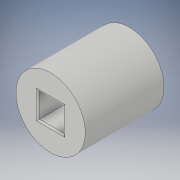
# Autodesk Inventor part: spline coupling
Saved by Autodesk Inventor 2017 (Build 210142000, 142)
## iProperties
Created: 2017-11-16
Part Number: spline coupling
Material: Generic
Document SubType Name: Modeling
Designer: Mitch
Density: 1 g/cm^3
Appearance: Default
Author: Mitch
Autodesk Inventor part; units mm, degrees
ref_plane "YZ Plane" through (0, 0, 0) normal (1, 0, 0) x (0, 1, 0)
ref_plane "XZ Plane" through (0, 0, 0) normal (0, 1, 0) x (-1, 0, 0)
ref_plane "XY Plane" through (0, 0, 0) normal (0, 0, 1) x (1, 0, 0)
sketch "Sketch1" plane through (0, 0, 0) normal (0, 0, 1) x (1, 0, 0)
  circle A0 centre (0, 0) radius 5.588
  dimension "d0" = 11.176
  constraints: 1 centre point, 1 coincident
  measures "d0" diameter of A0
extrude "Extrusion1" add sketch "Sketch1" along normal blind 12.7
sketch "Sketch2" plane through (0, 0, 0) normal (0, 0, -1) x (-1, 0, 0)
  circle A0 centre (0, 0.2754) radius 2.667
  line L0 (0.25, 2.9307) -> (0.0654, 3.4634)
  line L1 (0.0534, 3.4719) -> (-0.0534, 3.4719)
  line L2 (-0.0654, 3.4634) -> (-0.25, 2.9307)
  line L3 (0.25, 2.9307) -> (-0.25, 2.9307)
  line L4 (0, 4.3756) -> (0, 0.2754)
  arc A1 (-0.0534, 3.4719) -> (-0.0654, 3.4634) centre (-0.0534, 3.4592) ccw
  arc A2 (0.0654, 3.4634) -> (0.0534, 3.4719) centre (0.0534, 3.4592) ccw
  point P0 (0, 0)
  point P1 (0.0625, 3.4719)
  point P2 (-0.0625, 3.4719)
  dimension "d3" = 5.334
  dimension "d26" = 0.0625
  dimension "d27" = 0.0625
  dimension "d29" = 0.25
  dimension "d30" = 0.25
  dimension "d31" = 0.5413
  dimension "d32" = 0.0127
  constraints: 10 end point, 4 point on circle, 4 point on line, 4 tangent, 2 centre point, 1 equal radius, 1 horizontal, 1 parallel, 3 other
  measures "d26" distance from line of point (0.062, 3.472) L4
  measures "d27" distance from line of point (-0.062, 3.472) L4
  measures "d29" distance from line of L0.start L4
  measures "d30" distance from line of L2.end L4
  measures "d31" distance between parallel lines of L3 L1
  measures "d32" radius of A1
extrude "Extrusion2" cut sketch "Sketch2" against normal blind 3.81 contours A0 L3 | L3 L4 A0 | A0 L4 L3
sketch "Sketch3" plane through (0, 0, 0) normal (0, 0, -1) x (-1, 0, 0)
  circle A0 centre (0, 0.2754) radius 2.667 projected
  line L0 (0, 0.2754) -> (0, 5.2582)
  line L1 (-0.25, 2.9307) -> (-0.0625, 3.4719)
  line L2 (-0.0625, 3.4719) -> (0.0625, 3.4719)
  line L3 (0.0625, 3.4719) -> (0.25, 2.9307)
  line L4 (-0.25, 2.9307) -> (0.25, 2.9307)
  point P0 (0, 0)
  dimension "d35" = 0.0625
  dimension "d36" = 0.0625
  dimension "d37" = 0.25
  dimension "d38" = 0.5413
  constraints: 10 end point, 2 point on circle, 1 horizontal, 1 parallel, 1 vertical
  measures "d35" distance from line of L2.end L0
  measures "d36" distance from line of L1.end L0
  measures "d37" distance from line of L1.start L0
  measures "d38" distance between parallel lines of L4 L2
extrude "Extrusion3" cut sketch "Sketch3" against normal blind 3.81 contours A0 L0 L2 L3 | L1 L2 L0 A0
pattern_circular "Circular Pattern1" count 23 over 360 about axis through (0, 0.2754, 0) along (0, 0, 1) of "Extrusion3"
fillet "Fillet1" radius 0.254 23 edges at (-1.0625, 2.7216, 0) (-0.3632, 2.9176, 0) (0.3632, 2.9176, 0) (1.0625, 2.7216, 0) (1.6831, 2.3442, 0) (2.1789, 1.8134, 0) (2.513, 1.1685, 0) (2.6608, 0.4574, 0) (2.6112, -0.2672, 0) (2.368, -0.9516, 0) (1.9491, -1.545, 0) (1.3857, -2.0033, 0) (0.7195, -2.2927, 0) (0, -2.3916, 0) (-0.7195, -2.2927, 0) (-1.3857, -2.0033, 0) (-1.9491, -1.545, 0) (-2.368, -0.9516, 0) (-2.6112, -0.2672, 0) (-2.6608, 0.4574, 0) (-2.513, 1.1685, 0) (-2.1789, 1.8134, 0) (-1.6831, 2.3442, 0)
sketch "Sketch4" plane through (0, 0, 12.7) normal (0, 0, 1) x (1, 0, 0)
  line L0 (2.032, 2.032) -> (-2.032, 2.032)
  line L1 (-2.032, 2.032) -> (-2.032, -2.032)
  line L2 (-2.032, -2.032) -> (2.032, -2.032)
  line L3 (2.032, -2.032) -> (2.032, 2.032)
  constraints: 8 end point, 2 parallel, 1 horizontal, 1 perpendicular
extrude "Extrusion4" cut sketch "Sketch4" against normal blind 6.35
fillet "Fillet2" radius 0.254 4 edges at (0, 2.032, 12.7) (-2.032, 0, 12.7) (2.032, 0, 12.7) (0, -2.032, 12.7)
body "Solid1"
